Autodesk Fusion 360 part; units mm, degrees
(part 4 of 7)
sketch "Sketch3 (5)" plane through (0, 0, -1.1752) normal (0, 0, 1) x (-1, 0, 0)
  arc A0 (-21.9982, -2.8847) -> (-22.282, -3.9438) centre (-17.5834, -4.6352) ccw
  line L0 (-22.282, -3.9438) -> (-23.1617, -3.816)
  spline S0 degree 5 poles (-23.1617, -3.816) (-23.1657, -3.8154) (-23.1736, -3.8144) (-23.1855, -3.8132) (-23.2015, -3.8124) (-23.2215, -3.8123) (-23.2416, -3.8129) (-23.2618, -3.814) (-23.282, -3.8153) (-23.3022, -3.8168) (-23.3225, -3.8184) (-23.3427, -3.8203) (-23.363, -3.8225) (-23.3833, -3.825) (-23.4037, -3.8279) (-23.424, -3.8311) (-23.4444, -3.8346) (-23.4648, -3.8383) (-23.4852, -3.8422) (-23.5056, -3.8464) (-23.526, -3.8507) (-23.5464, -3.8552) (-23.5669, -3.86) (-23.5873, -3.865) (-23.6077, -3.8702) (-23.6282, -3.8756) (-23.6486, -3.8812) (-23.6691, -3.8871) (-23.6895, -3.8931) (-23.71, -3.8993) (-23.7304, -3.9057) (-23.7509, -3.9123) (-23.7713, -3.919) (-23.7917, -3.926) (-23.8122, -3.9331) (-23.8326, -3.9404) (-23.853, -3.9479) (-23.8734, -3.9556) (-23.8938, -3.9634) (-23.9142, -3.9714) (-23.9345, -3.9796) (-23.9549, -3.988) (-23.9753, -3.9965) (-23.9956, -4.0052) (-24.0159, -4.014) (-24.0362, -4.0231) (-24.0565, -4.0322) (-24.0768, -4.0416) (-24.0971, -4.0511) (-24.1173, -4.0607) (-24.1375, -4.0706) (-24.1577, -4.0805) (-24.1779, -4.0907) (-24.1981, -4.101) (-24.2182, -4.1114) (-24.2384, -4.122) (-24.2585, -4.1327) (-24.2785, -4.1436) (-24.2986, -4.1547) (-24.3186, -4.1659) (-24.3386, -4.1772) (-24.3586, -4.1887) (-24.3786, -4.2004) (-24.3985, -4.2122) (-24.4184, -4.2241) (-24.4383, -4.2362) (-24.4581, -4.2484) (-24.4779, -4.2608) (-24.4977, -4.2733) (-24.5174, -4.286) (-24.5372, -4.2988) (-24.5529, -4.3091) (-24.5647, -4.317) (-24.5726, -4.3222) (-24.5765, -4.3248) knots 0 0 0 0 0 0 0.01428571 0.02857143 0.04285714 0.05714286 0.07142857 0.08571429 0.1 0.11428571 0.12857143 0.14285714 0.15714286 0.17142857 0.18571429 0.2 0.21428571 0.22857143 0.24285714 0.25714286 0.27142857 0.28571429 0.3 0.31428571 0.32857143 0.34285714 0.35714286 0.37142857 0.38571429 0.4 0.41428571 0.42857143 0.44285714 0.45714286 0.47142857 0.48571429 0.5 0.51428571 0.52857143 0.54285714 0.55714286 0.57142857 0.58571429 0.6 0.61428571 0.62857143 0.64285714 0.65714286 0.67142857 0.68571429 0.7 0.71428571 0.72857143 0.74285714 0.75714286 0.77142857 0.78571429 0.8 0.81428571 0.82857143 0.84285714 0.85714286 0.87142857 0.88571429 0.9 0.91428571 0.92857143 0.94285714 0.95714286 0.97142857 0.98571429 1 1 1 1 1 1
  arc A1 (-24.5765, -4.3248) -> (-24.5765, -4.9455) centre (-17.5834, -4.6352) ccw
  spline S1 degree 5 poles (-24.5765, -4.9455) (-24.5726, -4.9482) (-24.5647, -4.9534) (-24.5529, -4.9612) (-24.5372, -4.9716) (-24.5174, -4.9844) (-24.4977, -4.997) (-24.4779, -5.0095) (-24.4581, -5.0219) (-24.4383, -5.0341) (-24.4184, -5.0462) (-24.3985, -5.0582) (-24.3786, -5.07) (-24.3586, -5.0816) (-24.3386, -5.0931) (-24.3186, -5.1044) (-24.2986, -5.1156) (-24.2785, -5.1267) (-24.2585, -5.1376) (-24.2384, -5.1483) (-24.2182, -5.1589) (-24.1981, -5.1694) (-24.1779, -5.1797) (-24.1577, -5.1898) (-24.1375, -5.1998) (-24.1173, -5.2096) (-24.0971, -5.2193) (-24.0768, -5.2288) (-24.0565, -5.2381) (-24.0362, -5.2473) (-24.0159, -5.2563) (-23.9956, -5.2652) (-23.9753, -5.2738) (-23.9549, -5.2824) (-23.9345, -5.2907) (-23.9142, -5.2989) (-23.8938, -5.3069) (-23.8734, -5.3148) (-23.853, -5.3224) (-23.8326, -5.3299) (-23.8122, -5.3372) (-23.7917, -5.3444) (-23.7713, -5.3513) (-23.7509, -5.3581) (-23.7304, -5.3647) (-23.71, -5.3711) (-23.6895, -5.3773) (-23.6691, -5.3833) (-23.6486, -5.3891) (-23.6282, -5.3947) (-23.6077, -5.4002) (-23.5873, -5.4054) (-23.5669, -5.4104) (-23.5464, -5.4151) (-23.526, -5.4197) (-23.5056, -5.424) (-23.4852, -5.4281) (-23.4648, -5.4321) (-23.4444, -5.4358) (-23.424, -5.4393) (-23.4037, -5.4425) (-23.3833, -5.4454) (-23.363, -5.4479) (-23.3427, -5.4501) (-23.3225, -5.4519) (-23.3022, -5.4536) (-23.282, -5.4551) (-23.2618, -5.4564) (-23.2416, -5.4574) (-23.2215, -5.458) (-23.2015, -5.458) (-23.1855, -5.4571) (-23.1736, -5.4559) (-23.1657, -5.4549) (-23.1617, -5.4543) knots -1 -1 -1 -1 -1 -1 -0.98571429 -0.97142857 -0.95714286 -0.94285714 -0.92857143 -0.91428571 -0.9 -0.88571429 -0.87142857 -0.85714286 -0.84285714 -0.82857143 -0.81428571 -0.8 -0.78571429 -0.77142857 -0.75714286 -0.74285714 -0.72857143 -0.71428571 -0.7 -0.68571429 -0.67142857 -0.65714286 -0.64285714 -0.62857143 -0.61428571 -0.6 -0.58571429 -0.57142857 -0.55714286 -0.54285714 -0.52857143 -0.51428571 -0.5 -0.48571429 -0.47142857 -0.45714286 -0.44285714 -0.42857143 -0.41428571 -0.4 -0.38571429 -0.37142857 -0.35714286 -0.34285714 -0.32857143 -0.31428571 -0.3 -0.28571429 -0.27142857 -0.25714286 -0.24285714 -0.22857143 -0.21428571 -0.2 -0.18571429 -0.17142857 -0.15714286 -0.14285714 -0.12857143 -0.11428571 -0.1 -0.08571429 -0.07142857 -0.05714286 -0.04285714 -0.02857143 -0.01428571 0 0 0 0 0 0
  line L1 (-23.1617, -5.4543) -> (-22.282, -5.3266)
  arc A2 (-22.282, -5.3266) -> (-21.9982, -6.3857) centre (-17.5834, -4.6352) ccw
  line L2 (-21.9982, -6.3857) -> (-22.8239, -6.7149)
  spline S2 degree 5 poles (-22.8239, -6.7149) (-22.8277, -6.7164) (-22.835, -6.7195) (-22.8459, -6.7244) (-22.8602, -6.7317) (-22.8776, -6.7416) (-22.8947, -6.7522) (-22.9116, -6.7632) (-22.9285, -6.7744) (-22.9452, -6.7858) (-22.9619, -6.7974) (-22.9786, -6.8091) (-22.995, -6.8212) (-23.0114, -6.8335) (-23.0275, -6.8462) (-23.0436, -6.8591) (-23.0595, -6.8723) (-23.0753, -6.8857) (-23.091, -6.8994) (-23.1066, -6.9131) (-23.1221, -6.9271) (-23.1375, -6.9412) (-23.1528, -6.9556) (-23.168, -6.9701) (-23.1831, -6.9849) (-23.1981, -6.9998) (-23.213, -7.0149) (-23.2278, -7.0301) (-23.2425, -7.0456) (-23.2571, -7.0612) (-23.2716, -7.0769) (-23.286, -7.0929) (-23.3003, -7.1089) (-23.3146, -7.1252) (-23.3287, -7.1416) (-23.3427, -7.1581) (-23.3566, -7.1748) (-23.3705, -7.1916) (-23.3842, -7.2086) (-23.3979, -7.2258) (-23.4114, -7.243) (-23.4249, -7.2605) (-23.4382, -7.278) (-23.4515, -7.2957) (-23.4647, -7.3135) (-23.4778, -7.3315) (-23.4907, -7.3496) (-23.5036, -7.3678) (-23.5164, -7.3862) (-23.5291, -7.4047) (-23.5417, -7.4233) (-23.5543, -7.442) (-23.5667, -7.4609) (-23.579, -7.4799) (-23.5912, -7.499) (-23.6033, -7.5182) (-23.6154, -7.5376) (-23.6273, -7.5571) (-23.6392, -7.5767) (-23.6509, -7.5964) (-23.6626, -7.6162) (-23.6741, -7.6362) (-23.6856, -7.6562) (-23.6969, -7.6764) (-23.7082, -7.6967) (-23.7194, -7.7171) (-23.7304, -7.7376) (-23.7414, -7.7582) (-23.7523, -7.7789) (-23.7631, -7.7998) (-23.7737, -7.8207) (-23.7822, -7.8376) (-23.7885, -7.8502) (-23.7927, -7.8587) (-23.7948, -7.863) knots 0 0 0 0 0 0 0.01428571 0.02857143 0.04285714 0.05714286 0.07142857 0.08571429 0.1 0.11428571 0.12857143 0.14285714 0.15714286 0.17142857 0.18571429 0.2 0.21428571 0.22857143 0.24285714 0.25714286 0.27142857 0.28571429 0.3 0.31428571 0.32857143 0.34285714 0.35714286 0.37142857 0.38571429 0.4 0.41428571 0.42857143 0.44285714 0.45714286 0.47142857 0.48571429 0.5 0.51428571 0.52857143 0.54285714 0.55714286 0.57142857 0.58571429 0.6 0.61428571 0.62857143 0.64285714 0.65714286 0.67142857 0.68571429 0.7 0.71428571 0.72857143 0.74285714 0.75714286 0.77142857 0.78571429 0.8 0.81428571 0.82857143 0.84285714 0.85714286 0.87142857 0.88571429 0.9 0.91428571 0.92857143 0.94285714 0.95714286 0.97142857 0.98571429 1 1 1 1 1 1
  arc A3 (-23.7948, -7.863) -> (-23.4844, -8.4005) centre (-17.5834, -4.6352) ccw
  spline S3 degree 5 poles (-23.4844, -8.4005) (-23.4797, -8.4008) (-23.4703, -8.4014) (-23.4561, -8.4023) (-23.4373, -8.4034) (-23.4139, -8.4046) (-23.3904, -8.4057) (-23.367, -8.4067) (-23.3437, -8.4075) (-23.3204, -8.4081) (-23.2971, -8.4087) (-23.2739, -8.409) (-23.2508, -8.4093) (-23.2277, -8.4094) (-23.2046, -8.4094) (-23.1816, -8.4092) (-23.1587, -8.4089) (-23.1358, -8.4084) (-23.113, -8.4078) (-23.0902, -8.4071) (-23.0674, -8.4062) (-23.0448, -8.4052) (-23.0222, -8.404) (-22.9996, -8.4027) (-22.9771, -8.4012) (-22.9547, -8.3996) (-22.9323, -8.3978) (-22.91, -8.3959) (-22.8878, -8.3939) (-22.8657, -8.3917) (-22.8436, -8.3894) (-22.8215, -8.3869) (-22.7996, -8.3842) (-22.7777, -8.3814) (-22.7559, -8.3785) (-22.7341, -8.3754) (-22.7125, -8.3721) (-22.6909, -8.3687) (-22.6694, -8.3652) (-22.648, -8.3614) (-22.6266, -8.3576) (-22.6054, -8.3535) (-22.5842, -8.3493) (-22.5631, -8.345) (-22.5421, -8.3404) (-22.5212, -8.3358) (-22.5004, -8.3309) (-22.4797, -8.3259) (-22.4591, -8.3207) (-22.4386, -8.3154) (-22.4181, -8.3099) (-22.3978, -8.3042) (-22.3776, -8.2983) (-22.3576, -8.2922) (-22.3376, -8.2859) (-22.3178, -8.2794) (-22.298, -8.2728) (-22.2784, -8.266) (-22.2589, -8.259) (-22.2395, -8.2519) (-22.2202, -8.2445) (-22.2012, -8.2368) (-22.1823, -8.2288) (-22.1637, -8.2206) (-22.1452, -8.2121) (-22.1268, -8.2034) (-22.1086, -8.1945) (-22.0904, -8.1856) (-22.0724, -8.1764) (-22.0547, -8.1669) (-22.0374, -8.1568) (-22.024, -8.1481) (-22.0143, -8.1411) (-22.0079, -8.1362) (-22.0048, -8.1338) knots -1 -1 -1 -1 -1 -1 -0.98571429 -0.97142857 -0.95714286 -0.94285714 -0.92857143 -0.91428571 -0.9 -0.88571429 -0.87142857 -0.85714286 -0.84285714 -0.82857143 -0.81428571 -0.8 -0.78571429 -0.77142857 -0.75714286 -0.74285714 -0.72857143 -0.71428571 -0.7 -0.68571429 -0.67142857 -0.65714286 -0.64285714 -0.62857143 -0.61428571 -0.6 -0.58571429 -0.57142857 -0.55714286 -0.54285714 -0.52857143 -0.51428571 -0.5 -0.48571429 -0.47142857 -0.45714286 -0.44285714 -0.42857143 -0.41428571 -0.4 -0.38571429 -0.37142857 -0.35714286 -0.34285714 -0.32857143 -0.31428571 -0.3 -0.28571429 -0.27142857 -0.25714286 -0.24285714 -0.22857143 -0.21428571 -0.2 -0.18571429 -0.17142857 -0.15714286 -0.14285714 -0.12857143 -0.11428571 -0.1 -0.08571429 -0.07142857 -0.05714286 -0.04285714 -0.02857143 -0.01428571 0 0 0 0 0 0
  line L3 (-22.0048, -8.1338) -> (-21.3068, -7.5833)
  arc A4 (-21.3068, -7.5833) -> (-20.5315, -8.3586) centre (-17.5834, -4.6352) ccw
  line L4 (-20.5315, -8.3586) -> (-21.082, -9.0566)
  spline S4 degree 5 poles (-21.082, -9.0566) (-21.0844, -9.0597) (-21.0893, -9.0661) (-21.0963, -9.0758) (-21.105, -9.0892) (-21.1151, -9.1065) (-21.1246, -9.1242) (-21.1338, -9.1422) (-21.1427, -9.1604) (-21.1516, -9.1786) (-21.1603, -9.197) (-21.1688, -9.2155) (-21.177, -9.2341) (-21.185, -9.253) (-21.1927, -9.272) (-21.2001, -9.2913) (-21.2072, -9.3107) (-21.2142, -9.3302) (-21.221, -9.3498) (-21.2276, -9.3696) (-21.2341, -9.3894) (-21.2404, -9.4094) (-21.2465, -9.4294) (-21.2524, -9.4496) (-21.2581, -9.4699) (-21.2636, -9.4903) (-21.2689, -9.5109) (-21.2741, -9.5315) (-21.2791, -9.5522) (-21.284, -9.573) (-21.2887, -9.5939) (-21.2932, -9.6149) (-21.2975, -9.636) (-21.3017, -9.6572) (-21.3058, -9.6784) (-21.3096, -9.6998) (-21.3134, -9.7212) (-21.3169, -9.7427) (-21.3203, -9.7643) (-21.3236, -9.7859) (-21.3267, -9.8077) (-21.3296, -9.8295) (-21.3324, -9.8514) (-21.3351, -9.8733) (-21.3376, -9.8953) (-21.3399, -9.9174) (-21.3421, -9.9396) (-21.3442, -9.9618) (-21.3461, -9.9841) (-21.3478, -10.0065) (-21.3494, -10.0289) (-21.3509, -10.0514) (-21.3522, -10.074) (-21.3534, -10.0966) (-21.3544, -10.1192) (-21.3553, -10.142) (-21.356, -10.1647) (-21.3566, -10.1876) (-21.3571, -10.2105) (-21.3574, -10.2334) (-21.3576, -10.2564) (-21.3576, -10.2795) (-21.3575, -10.3026) (-21.3573, -10.3257) (-21.3569, -10.3489) (-21.3563, -10.3722) (-21.3557, -10.3955) (-21.3549, -10.4188) (-21.3539, -10.4422) (-21.3528, -10.4656) (-21.3516, -10.4891) (-21.3505, -10.5079) (-21.3496, -10.5221) (-21.349, -10.5315) (-21.3487, -10.5362) knots 0 0 0 0 0 0 0.01428571 0.02857143 0.04285714 0.05714286 0.07142857 0.08571429 0.1 0.11428571 0.12857143 0.14285714 0.15714286 0.17142857 0.18571429 0.2 0.21428571 0.22857143 0.24285714 0.25714286 0.27142857 0.28571429 0.3 0.31428571 0.32857143 0.34285714 0.35714286 0.37142857 0.38571429 0.4 0.41428571 0.42857143 0.44285714 0.45714286 0.47142857 0.48571429 0.5 0.51428571 0.52857143 0.54285714 0.55714286 0.57142857 0.58571429 0.6 0.61428571 0.62857143 0.64285714 0.65714286 0.67142857 0.68571429 0.7 0.71428571 0.72857143 0.74285714 0.75714286 0.77142857 0.78571429 0.8 0.81428571 0.82857143 0.84285714 0.85714286 0.87142857 0.88571429 0.9 0.91428571 0.92857143 0.94285714 0.95714286 0.97142857 0.98571429 1 1 1 1 1 1
  arc A5 (-21.3487, -10.5362) -> (-20.8112, -10.8466) centre (-17.5834, -4.6352) ccw
  spline S5 degree 5 poles (-20.8112, -10.8466) (-20.8069, -10.8445) (-20.7985, -10.8403) (-20.7858, -10.834) (-20.7689, -10.8255) (-20.748, -10.8148) (-20.7272, -10.8041) (-20.7064, -10.7932) (-20.6858, -10.7822) (-20.6653, -10.7712) (-20.6449, -10.76) (-20.6246, -10.7487) (-20.6044, -10.7374) (-20.5844, -10.7259) (-20.5644, -10.7143) (-20.5446, -10.7027) (-20.5249, -10.6909) (-20.5053, -10.6791) (-20.4858, -10.6672) (-20.4664, -10.6551) (-20.4472, -10.643) (-20.4281, -10.6308) (-20.4091, -10.6185) (-20.3902, -10.606) (-20.3715, -10.5935) (-20.3529, -10.5809) (-20.3344, -10.5682) (-20.316, -10.5554) (-20.2978, -10.5425) (-20.2797, -10.5296) (-20.2617, -10.5165) (-20.2439, -10.5033) (-20.2262, -10.49) (-20.2087, -10.4767) (-20.1912, -10.4632) (-20.174, -10.4497) (-20.1568, -10.436) (-20.1398, -10.4223) (-20.123, -10.4084) (-20.1063, -10.3945) (-20.0898, -10.3805) (-20.0734, -10.3664) (-20.0571, -10.3521) (-20.0411, -10.3378) (-20.0251, -10.3234) (-20.0094, -10.3089) (-19.9938, -10.2943) (-19.9784, -10.2796) (-19.9631, -10.2648) (-19.948, -10.2499) (-19.9331, -10.2349) (-19.9183, -10.2198) (-19.9038, -10.2046) (-19.8895, -10.1893) (-19.8753, -10.1739) (-19.8613, -10.1584) (-19.8476, -10.1428) (-19.834, -10.1271) (-19.8205, -10.1113) (-19.8073, -10.0954) (-19.7944, -10.0793) (-19.7817, -10.0632) (-19.7694, -10.0468) (-19.7573, -10.0304) (-19.7456, -10.0137) (-19.734, -9.997) (-19.7226, -9.9803) (-19.7114, -9.9634) (-19.7004, -9.9465) (-19.6898, -9.9294) (-19.6799, -9.912) (-19.6726, -9.8977) (-19.6677, -9.8868) (-19.6646, -9.8794) (-19.6631, -9.8757) knots -1 -1 -1 -1 -1 -1 -0.98571429 -0.97142857 -0.95714286 -0.94285714 -0.92857143 -0.91428571 -0.9 -0.88571429 -0.87142857 -0.85714286 -0.84285714 -0.82857143 -0.81428571 -0.8 -0.78571429 -0.77142857 -0.75714286 -0.74285714 -0.72857143 -0.71428571 -0.7 -0.68571429 -0.67142857 -0.65714286 -0.64285714 -0.62857143 -0.61428571 -0.6 -0.58571429 -0.57142857 -0.55714286 -0.54285714 -0.52857143 -0.51428571 -0.5 -0.48571429 -0.47142857 -0.45714286 -0.44285714 -0.42857143 -0.41428571 -0.4 -0.38571429 -0.37142857 -0.35714286 -0.34285714 -0.32857143 -0.31428571 -0.3 -0.28571429 -0.27142857 -0.25714286 -0.24285714 -0.22857143 -0.21428571 -0.2 -0.18571429 -0.17142857 -0.15714286 -0.14285714 -0.12857143 -0.11428571 -0.1 -0.08571429 -0.07142857 -0.05714286 -0.04285714 -0.02857143 -0.01428571 0 0 0 0 0 0
  line L5 (-19.6631, -9.8757) -> (-19.3339, -9.05)
  arc A6 (-19.3339, -9.05) -> (-18.2748, -9.3338) centre (-17.5834, -4.6352) ccw
  line L6 (-18.2748, -9.3338) -> (-18.4025, -10.2135)
  spline S6 degree 5 poles (-18.4025, -10.2135) (-18.4031, -10.2175) (-18.4041, -10.2254) (-18.4053, -10.2373) (-18.4062, -10.2533) (-18.4063, -10.2733) (-18.4056, -10.2934) (-18.4046, -10.3136) (-18.4033, -10.3338) (-18.4018, -10.354) (-18.4001, -10.3742) (-18.3983, -10.3945) (-18.3961, -10.4148) (-18.3936, -10.4351) (-18.3907, -10.4555) (-18.3875, -10.4758) (-18.384, -10.4962) (-18.3803, -10.5166) (-18.3763, -10.537) (-18.3722, -10.5574) (-18.3679, -10.5778) (-18.3633, -10.5982) (-18.3586, -10.6187) (-18.3536, -10.6391) (-18.3484, -10.6595) (-18.343, -10.68) (-18.3373, -10.7004) (-18.3315, -10.7209) (-18.3255, -10.7413) (-18.3193, -10.7618) (-18.3129, -10.7822) (-18.3063, -10.8027) (-18.2995, -10.8231) (-18.2926, -10.8435) (-18.2854, -10.8639) (-18.2781, -10.8844) (-18.2706, -10.9048) (-18.263, -10.9252) (-18.2551, -10.9456) (-18.2471, -10.966) (-18.2389, -10.9863) (-18.2306, -11.0067) (-18.2221, -11.027) (-18.2134, -11.0474) (-18.2045, -11.0677) (-18.1955, -11.088) (-18.1863, -11.1083) (-18.177, -11.1286) (-18.1675, -11.1488) (-18.1578, -11.1691) (-18.148, -11.1893) (-18.138, -11.2095) (-18.1279, -11.2297) (-18.1176, -11.2499) (-18.1072, -11.27) (-18.0966, -11.2901) (-18.0858, -11.3102) (-18.0749, -11.3303) (-18.0639, -11.3504) (-18.0527, -11.3704) (-18.0413, -11.3904) (-18.0298, -11.4104) (-18.0182, -11.4303) (-18.0064, -11.4503) (-17.9944, -11.4702) (-17.9824, -11.49) (-17.9701, -11.5099) (-17.9578, -11.5297) (-17.9452, -11.5495) (-17.9326, -11.5692) (-17.9198, -11.589) (-17.9094, -11.6047) (-17.9016, -11.6165) (-17.8964, -11.6244) (-17.8937, -11.6283) knots 0 0 0 0 0 0 0.01428571 0.02857143 0.04285714 0.05714286 0.07142857 0.08571429 0.1 0.11428571 0.12857143 0.14285714 0.15714286 0.17142857 0.18571429 0.2 0.21428571 0.22857143 0.24285714 0.25714286 0.27142857 0.28571429 0.3 0.31428571 0.32857143 0.34285714 0.35714286 0.37142857 0.38571429 0.4 0.41428571 0.42857143 0.44285714 0.45714286 0.47142857 0.48571429 0.5 0.51428571 0.52857143 0.54285714 0.55714286 0.57142857 0.58571429 0.6 0.61428571 0.62857143 0.64285714 0.65714286 0.67142857 0.68571429 0.7 0.71428571 0.72857143 0.74285714 0.75714286 0.77142857 0.78571429 0.8 0.81428571 0.82857143 0.84285714 0.85714286 0.87142857 0.88571429 0.9 0.91428571 0.92857143 0.94285714 0.95714286 0.97142857 0.98571429 1 1 1 1 1 1
  arc A7 (-17.8937, -11.6283) -> (-17.273, -11.6283) centre (-17.5834, -4.6352) ccw
  spline S7 degree 5 poles (-17.273, -11.6283) (-17.2704, -11.6244) (-17.2652, -11.6165) (-17.2573, -11.6047) (-17.247, -11.589) (-17.2342, -11.5692) (-17.2215, -11.5495) (-17.209, -11.5297) (-17.1966, -11.5099) (-17.1844, -11.49) (-17.1723, -11.4702) (-17.1604, -11.4503) (-17.1486, -11.4303) (-17.137, -11.4104) (-17.1255, -11.3904) (-17.1141, -11.3704) (-17.1029, -11.3504) (-17.0919, -11.3303) (-17.081, -11.3102) (-17.0702, -11.2901) (-17.0596, -11.27) (-17.0492, -11.2499) (-17.0389, -11.2297) (-17.0288, -11.2095) (-17.0188, -11.1893) (-17.009, -11.1691) (-16.9993, -11.1488) (-16.9898, -11.1286) (-16.9804, -11.1083) (-16.9713, -11.088) (-16.9623, -11.0677) (-16.9534, -11.0474) (-16.9447, -11.027) (-16.9362, -11.0067) (-16.9278, -10.9863) (-16.9197, -10.966) (-16.9116, -10.9456) (-16.9038, -10.9252) (-16.8961, -10.9048) (-16.8886, -10.8844) (-16.8813, -10.8639) (-16.8742, -10.8435) (-16.8672, -10.8231) (-16.8605, -10.8027) (-16.8539, -10.7822) (-16.8475, -10.7618) (-16.8413, -10.7413) (-16.8353, -10.7209) (-16.8294, -10.7004) (-16.8238, -10.68) (-16.8184, -10.6595) (-16.8132, -10.6391) (-16.8082, -10.6187) (-16.8034, -10.5982) (-16.7989, -10.5778) (-16.7946, -10.5574) (-16.7904, -10.537) (-16.7865, -10.5166) (-16.7828, -10.4962) (-16.7793, -10.4758) (-16.7761, -10.4555) (-16.7732, -10.4351) (-16.7707, -10.4148) (-16.7685, -10.3945) (-16.7666, -10.3742) (-16.765, -10.354) (-16.7635, -10.3338) (-16.7622, -10.3136) (-16.7611, -10.2934) (-16.7605, -10.2733) (-16.7606, -10.2533) (-16.7615, -10.2373) (-16.7626, -10.2254) (-16.7637, -10.2175) (-16.7642, -10.2135) knots -1 -1 -1 -1 -1 -1 -0.98571429 -0.97142857 -0.95714286 -0.94285714 -0.92857143 -0.91428571 -0.9 -0.88571429 -0.87142857 -0.85714286 -0.84285714 -0.82857143 -0.81428571 -0.8 -0.78571429 -0.77142857 -0.75714286 -0.74285714 -0.72857143 -0.71428571 -0.7 -0.68571429 -0.67142857 -0.65714286 -0.64285714 -0.62857143 -0.61428571 -0.6 -0.58571429 -0.57142857 -0.55714286 -0.54285714 -0.52857143 -0.51428571 -0.5 -0.48571429 -0.47142857 -0.45714286 -0.44285714 -0.42857143 -0.41428571 -0.4 -0.38571429 -0.37142857 -0.35714286 -0.34285714 -0.32857143 -0.31428571 -0.3 -0.28571429 -0.27142857 -0.25714286 -0.24285714 -0.22857143 -0.21428571 -0.2 -0.18571429 -0.17142857 -0.15714286 -0.14285714 -0.12857143 -0.11428571 -0.1 -0.08571429 -0.07142857 -0.05714286 -0.04285714 -0.02857143 -0.01428571 0 0 0 0 0 0
  line L7 (-16.7642, -10.2135) -> (-16.892, -9.3338)
  arc A8 (-16.892, -9.3338) -> (-15.8329, -9.05) centre (-17.5834, -4.6352) ccw
  line L8 (-15.8329, -9.05) -> (-15.5036, -9.8757)
  spline S8 degree 5 poles (-15.5036, -9.8757) (-15.5021, -9.8794) (-15.4991, -9.8868) (-15.4941, -9.8977) (-15.4869, -9.912) (-15.4769, -9.9294) (-15.4663, -9.9465) (-15.4554, -9.9634) (-15.4441, -9.9803) (-15.4327, -9.997) (-15.4212, -10.0137) (-15.4094, -10.0304) (-15.3974, -10.0468) (-15.385, -10.0632) (-15.3724, -10.0793) (-15.3594, -10.0954) (-15.3462, -10.1113) (-15.3328, -10.1271) (-15.3192, -10.1428) (-15.3054, -10.1584) (-15.2915, -10.1739) (-15.2773, -10.1893) (-15.263, -10.2046) (-15.2484, -10.2198) (-15.2337, -10.2349) (-15.2188, -10.2499) (-15.2037, -10.2648) (-15.1884, -10.2796) (-15.173, -10.2943) (-15.1574, -10.3089) (-15.1416, -10.3234) (-15.1257, -10.3378) (-15.1096, -10.3521) (-15.0934, -10.3664) (-15.077, -10.3805) (-15.0605, -10.3945) (-15.0438, -10.4084) (-15.0269, -10.4223) (-15.0099, -10.436) (-14.9928, -10.4497) (-14.9755, -10.4632) (-14.9581, -10.4767) (-14.9406, -10.49) (-14.9229, -10.5033) (-14.905, -10.5165) (-14.8871, -10.5296) (-14.869, -10.5425) (-14.8507, -10.5554) (-14.8324, -10.5682) (-14.8139, -10.5809) (-14.7953, -10.5935) (-14.7765, -10.606) (-14.7577, -10.6185) (-14.7387, -10.6308) (-14.7196, -10.643) (-14.7003, -10.6551) (-14.681, -10.6672) (-14.6615, -10.6791) (-14.6419, -10.6909) (-14.6222, -10.7027) (-14.6023, -10.7143) (-14.5824, -10.7259) (-14.5623, -10.7374) (-14.5422, -10.7487) (-14.5219, -10.76) (-14.5015, -10.7712) (-14.481, -10.7822) (-14.4603, -10.7932) (-14.4396, -10.8041) (-14.4188, -10.8148) (-14.3978, -10.8255) (-14.381, -10.834) (-14.3683, -10.8403) (-14.3598, -10.8445) (-14.3556, -10.8466) knots 0 0 0 0 0 0 0.01428571 0.02857143 0.04285714 0.05714286 0.07142857 0.08571429 0.1 0.11428571 0.12857143 0.14285714 0.15714286 0.17142857 0.18571429 0.2 0.21428571 0.22857143 0.24285714 0.25714286 0.27142857 0.28571429 0.3 0.31428571 0.32857143 0.34285714 0.35714286 0.37142857 0.38571429 0.4 0.41428571 0.42857143 0.44285714 0.45714286 0.47142857 0.48571429 0.5 0.51428571 0.52857143 0.54285714 0.55714286 0.57142857 0.58571429 0.6 0.61428571 0.62857143 0.64285714 0.65714286 0.67142857 0.68571429 0.7 0.71428571 0.72857143 0.74285714 0.75714286 0.77142857 0.78571429 0.8 0.81428571 0.82857143 0.84285714 0.85714286 0.87142857 0.88571429 0.9 0.91428571 0.92857143 0.94285714 0.95714286 0.97142857 0.98571429 1 1 1 1 1 1
  arc A9 (-14.3556, -10.8466) -> (-13.8181, -10.5362) centre (-17.5834, -4.6352) ccw
  spline S9 degree 5 poles (-13.8181, -10.5362) (-13.8177, -10.5315) (-13.8171, -10.5221) (-13.8162, -10.5079) (-13.8152, -10.4891) (-13.8139, -10.4656) (-13.8129, -10.4422) (-13.8119, -10.4188) (-13.8111, -10.3955) (-13.8104, -10.3722) (-13.8099, -10.3489) (-13.8095, -10.3257) (-13.8093, -10.3026) (-13.8092, -10.2795) (-13.8092, -10.2564) (-13.8094, -10.2334) (-13.8097, -10.2105) (-13.8101, -10.1876) (-13.8107, -10.1647) (-13.8115, -10.142) (-13.8124, -10.1192) (-13.8134, -10.0966) (-13.8146, -10.074) (-13.8159, -10.0514) (-13.8173, -10.0289) (-13.819, -10.0065) (-13.8207, -9.9841) (-13.8226, -9.9618) (-13.8247, -9.9396) (-13.8269, -9.9174) (-13.8292, -9.8953) (-13.8317, -9.8733) (-13.8343, -9.8514) (-13.8371, -9.8295) (-13.8401, -9.8077) (-13.8432, -9.7859) (-13.8464, -9.7643) (-13.8498, -9.7427) (-13.8534, -9.7212) (-13.8571, -9.6998) (-13.861, -9.6784) (-13.865, -9.6572) (-13.8692, -9.636) (-13.8736, -9.6149) (-13.8781, -9.5939) (-13.8828, -9.573) (-13.8876, -9.5522) (-13.8927, -9.5315) (-13.8978, -9.5109) (-13.9032, -9.4903) (-13.9087, -9.4699) (-13.9144, -9.4496) (-13.9203, -9.4294) (-13.9264, -9.4094) (-13.9327, -9.3894) (-13.9391, -9.3696) (-13.9458, -9.3498) (-13.9526, -9.3302) (-13.9595, -9.3107) (-13.9667, -9.2913) (-13.9741, -9.272) (-13.9818, -9.253) (-13.9897, -9.2341) (-13.998, -9.2155) (-14.0065, -9.197) (-14.0152, -9.1786) (-14.024, -9.1604) (-14.033, -9.1422) (-14.0422, -9.1242) (-14.0517, -9.1065) (-14.0618, -9.0892) (-14.0705, -9.0758) (-14.0775, -9.0661) (-14.0823, -9.0597) (-14.0848, -9.0566) knots -1 -1 -1 -1 -1 -1 -0.98571429 -0.97142857 -0.95714286 -0.94285714 -0.92857143 -0.91428571 -0.9 -0.88571429 -0.87142857 -0.85714286 -0.84285714 -0.82857143 -0.81428571 -0.8 -0.78571429 -0.77142857 -0.75714286 -0.74285714 -0.72857143 -0.71428571 -0.7 -0.68571429 -0.67142857 -0.65714286 -0.64285714 -0.62857143 -0.61428571 -0.6 -0.58571429 -0.57142857 -0.55714286 -0.54285714 -0.52857143 -0.51428571 -0.5 -0.48571429 -0.47142857 -0.45714286 -0.44285714 -0.42857143 -0.41428571 -0.4 -0.38571429 -0.37142857 -0.35714286 -0.34285714 -0.32857143 -0.31428571 -0.3 -0.28571429 -0.27142857 -0.25714286 -0.24285714 -0.22857143 -0.21428571 -0.2 -0.18571429 -0.17142857 -0.15714286 -0.14285714 -0.12857143 -0.11428571 -0.1 -0.08571429 -0.07142857 -0.05714286 -0.04285714 -0.02857143 -0.01428571 0 0 0 0 0 0
  line L9 (-14.0848, -9.0566) -> (-14.6353, -8.3586)
  arc A10 (-14.6353, -8.3586) -> (-13.86, -7.5833) centre (-17.5834, -4.6352) ccw
  line L10 (-13.86, -7.5833) -> (-13.162, -8.1338)
  spline S10 degree 5 poles (-13.162, -8.1338) (-13.1588, -8.1362) (-13.1525, -8.1411) (-13.1427, -8.1481) (-13.1293, -8.1568) (-13.112, -8.1669) (-13.0943, -8.1764) (-13.0763, -8.1856) (-13.0582, -8.1945) (-13.0399, -8.2034) (-13.0216, -8.2121) (-13.0031, -8.2206) (-12.9844, -8.2288) (-12.9656, -8.2368) (-12.9465, -8.2445) (-12.9273, -8.2519) (-12.9079, -8.259) (-12.8884, -8.266) (-12.8687, -8.2728) (-12.849, -8.2794) (-12.8292, -8.2859) (-12.8092, -8.2922) (-12.7891, -8.2983) (-12.7689, -8.3042) (-12.7486, -8.3099) (-12.7282, -8.3154) (-12.7077, -8.3207) (-12.6871, -8.3259) (-12.6663, -8.3309) (-12.6455, -8.3358) (-12.6246, -8.3404) (-12.6036, -8.345) (-12.5826, -8.3493) (-12.5614, -8.3535) (-12.5401, -8.3576) (-12.5188, -8.3614) (-12.4974, -8.3652) (-12.4759, -8.3687) (-12.4543, -8.3721) (-12.4326, -8.3754) (-12.4109, -8.3785) (-12.3891, -8.3814) (-12.3672, -8.3842) (-12.3452, -8.3869) (-12.3232, -8.3894) (-12.3011, -8.3917) (-12.279, -8.3939) (-12.2567, -8.3959) (-12.2344, -8.3978) (-12.2121, -8.3996) (-12.1896, -8.4012) (-12.1671, -8.4027) (-12.1446, -8.404) (-12.122, -8.4052) (-12.0993, -8.4062) (-12.0766, -8.4071) (-12.0538, -8.4078) (-12.031, -8.4084) (-12.0081, -8.4089) (-11.9851, -8.4092) (-11.9621, -8.4094) (-11.9391, -8.4094) (-11.916, -8.4093) (-11.8928, -8.409) (-11.8696, -8.4087) (-11.8464, -8.4081) (-11.8231, -8.4075) (-11.7997, -8.4067) (-11.7763, -8.4057) (-11.7529, -8.4046) (-11.7294, -8.4034) (-11.7106, -8.4023) (-11.6965, -8.4014) (-11.6871, -8.4008) (-11.6823, -8.4005) knots 0 0 0 0 0 0 0.01428571 0.02857143 0.04285714 0.05714286 0.07142857 0.08571429 0.1 0.11428571 0.12857143 0.14285714 0.15714286 0.17142857 0.18571429 0.2 0.21428571 0.22857143 0.24285714 0.25714286 0.27142857 0.28571429 0.3 0.31428571 0.32857143 0.34285714 0.35714286 0.37142857 0.38571429 0.4 0.41428571 0.42857143 0.44285714 0.45714286 0.47142857 0.48571429 0.5 0.51428571 0.52857143 0.54285714 0.55714286 0.57142857 0.58571429 0.6 0.61428571 0.62857143 0.64285714 0.65714286 0.67142857 0.68571429 0.7 0.71428571 0.72857143 0.74285714 0.75714286 0.77142857 0.78571429 0.8 0.81428571 0.82857143 0.84285714 0.85714286 0.87142857 0.88571429 0.9 0.91428571 0.92857143 0.94285714 0.95714286 0.97142857 0.98571429 1 1 1 1 1 1
  arc A11 (-11.6823, -8.4005) -> (-11.372, -7.863) centre (-17.5834, -4.6352) ccw
  spline S11 degree 5 poles (-11.372, -7.863) (-11.3741, -7.8587) (-11.3783, -7.8502) (-11.3846, -7.8376) (-11.393, -7.8207) (-11.4037, -7.7998) (-11.4145, -7.7789) (-11.4254, -7.7582) (-11.4363, -7.7376) (-11.4474, -7.7171) (-11.4586, -7.6967) (-11.4698, -7.6764) (-11.4812, -7.6562) (-11.4927, -7.6362) (-11.5042, -7.6162) (-11.5159, -7.5964) (-11.5276, -7.5767) (-11.5395, -7.5571) (-11.5514, -7.5376) (-11.5634, -7.5182) (-11.5756, -7.499) (-11.5878, -7.4799) (-11.6001, -7.4609) (-11.6125, -7.442) (-11.625, -7.4233) (-11.6376, -7.4047) (-11.6503, -7.3862) (-11.6631, -7.3678) (-11.676, -7.3496) (-11.689, -7.3315) (-11.7021, -7.3135) (-11.7153, -7.2957) (-11.7285, -7.278) (-11.7419, -7.2605) (-11.7553, -7.243) (-11.7689, -7.2258) (-11.7825, -7.2086) (-11.7963, -7.1916) (-11.8101, -7.1748) (-11.8241, -7.1581) (-11.8381, -7.1416) (-11.8522, -7.1252) (-11.8664, -7.1089) (-11.8807, -7.0929) (-11.8952, -7.0769) (-11.9097, -7.0612) (-11.9243, -7.0456) (-11.939, -7.0301) (-11.9538, -7.0149) (-11.9686, -6.9998) (-11.9836, -6.9849) (-11.9987, -6.9701) (-12.0139, -6.9556) (-12.0293, -6.9412) (-12.0447, -6.9271) (-12.0602, -6.9131) (-12.0758, -6.8994) (-12.0915, -6.8857) (-12.1073, -6.8723) (-12.1232, -6.8591) (-12.1392, -6.8462) (-12.1554, -6.8335) (-12.1717, -6.8212) (-12.1882, -6.8091) (-12.2048, -6.7974) (-12.2215, -6.7858) (-12.2383, -6.7744) (-12.2551, -6.7632) (-12.2721, -6.7522) (-12.2892, -6.7416) (-12.3066, -6.7317) (-12.3208, -6.7244) (-12.3317, -6.7195) (-12.3391, -6.7164) (-12.3428, -6.7149) knots -1 -1 -1 -1 -1 -1 -0.98571429 -0.97142857 -0.95714286 -0.94285714 -0.92857143 -0.91428571 -0.9 -0.88571429 -0.87142857 -0.85714286 -0.84285714 -0.82857143 -0.81428571 -0.8 -0.78571429 -0.77142857 -0.75714286 -0.74285714 -0.72857143 -0.71428571 -0.7 -0.68571429 -0.67142857 -0.65714286 -0.64285714 -0.62857143 -0.61428571 -0.6 -0.58571429 -0.57142857 -0.55714286 -0.54285714 -0.52857143 -0.51428571 -0.5 -0.48571429 -0.47142857 -0.45714286 -0.44285714 -0.42857143 -0.41428571 -0.4 -0.38571429 -0.37142857 -0.35714286 -0.34285714 -0.32857143 -0.31428571 -0.3 -0.28571429 -0.27142857 -0.25714286 -0.24285714 -0.22857143 -0.21428571 -0.2 -0.18571429 -0.17142857 -0.15714286 -0.14285714 -0.12857143 -0.11428571 -0.1 -0.08571429 -0.07142857 -0.05714286 -0.04285714 -0.02857143 -0.01428571 0 0 0 0 0 0
  line L11 (-12.3428, -6.7149) -> (-13.1686, -6.3857)
  arc A12 (-13.1686, -6.3857) -> (-12.8848, -5.3266) centre (-17.5834, -4.6352) ccw
  line L12 (-12.8848, -5.3266) -> (-12.0051, -5.4543)
  spline S12 degree 5 poles (-12.0051, -5.4543) (-12.0011, -5.4549) (-11.9932, -5.4559) (-11.9812, -5.4571) (-11.9653, -5.458) (-11.9452, -5.458) (-11.9251, -5.4574) (-11.905, -5.4564) (-11.8848, -5.4551) (-11.8646, -5.4536) (-11.8443, -5.4519) (-11.824, -5.4501) (-11.8038, -5.4479) (-11.7834, -5.4454) (-11.7631, -5.4425) (-11.7427, -5.4393) (-11.7224, -5.4358) (-11.702, -5.4321) (-11.6816, -5.4281) (-11.6612, -5.424) (-11.6408, -5.4197) (-11.6203, -5.4151) (-11.5999, -5.4104) (-11.5795, -5.4054) (-11.559, -5.4002) (-11.5386, -5.3947) (-11.5181, -5.3891) (-11.4977, -5.3833) (-11.4772, -5.3773) (-11.4568, -5.3711) (-11.4363, -5.3647) (-11.4159, -5.3581) (-11.3955, -5.3513) (-11.375, -5.3444) (-11.3546, -5.3372) (-11.3342, -5.3299) (-11.3138, -5.3224) (-11.2934, -5.3148) (-11.273, -5.3069) (-11.2526, -5.2989) (-11.2322, -5.2907) (-11.2119, -5.2824) (-11.1915, -5.2738) (-11.1712, -5.2652) (-11.1509, -5.2563) (-11.1305, -5.2473) (-11.1102, -5.2381) (-11.09, -5.2288) (-11.0697, -5.2193) (-11.0495, -5.2096) (-11.0292, -5.1998) (-11.009, -5.1898) (-10.9888, -5.1797) (-10.9687, -5.1694) (-10.9485, -5.1589) (-10.9284, -5.1483) (-10.9083, -5.1376) (-10.8882, -5.1267) (-10.8682, -5.1156) (-10.8481, -5.1044) (-10.8281, -5.0931) (-10.8082, -5.0816) (-10.7882, -5.07) (-10.7683, -5.0582) (-10.7484, -5.0462) (-10.7285, -5.0341) (-10.7087, -5.0219) (-10.6889, -5.0095) (-10.6691, -4.997) (-10.6493, -4.9844) (-10.6296, -4.9716) (-10.6139, -4.9612) (-10.6021, -4.9534) (-10.5942, -4.9482) (-10.5903, -4.9455) knots 0 0 0 0 0 0 0.01428571 0.02857143 0.04285714 0.05714286 0.07142857 0.08571429 0.1 0.11428571 0.12857143 0.14285714 0.15714286 0.17142857 0.18571429 0.2 0.21428571 0.22857143 0.24285714 0.25714286 0.27142857 0.28571429 0.3 0.31428571 0.32857143 0.34285714 0.35714286 0.37142857 0.38571429 0.4 0.41428571 0.42857143 0.44285714 0.45714286 0.47142857 0.48571429 0.5 0.51428571 0.52857143 0.54285714 0.55714286 0.57142857 0.58571429 0.6 0.61428571 0.62857143 0.64285714 0.65714286 0.67142857 0.68571429 0.7 0.71428571 0.72857143 0.74285714 0.75714286 0.77142857 0.78571429 0.8 0.81428571 0.82857143 0.84285714 0.85714286 0.87142857 0.88571429 0.9 0.91428571 0.92857143 0.94285714 0.95714286 0.97142857 0.98571429 1 1 1 1 1 1
  arc A13 (-10.5903, -4.9455) -> (-10.5903, -4.3248) centre (-17.5834, -4.6352) ccw
  spline S13 degree 5 poles (-10.5903, -4.3248) (-10.5942, -4.3222) (-10.6021, -4.317) (-10.6139, -4.3091) (-10.6296, -4.2988) (-10.6493, -4.286) (-10.6691, -4.2733) (-10.6889, -4.2608) (-10.7087, -4.2484) (-10.7285, -4.2362) (-10.7484, -4.2241) (-10.7683, -4.2122) (-10.7882, -4.2004) (-10.8082, -4.1887) (-10.8281, -4.1772) (-10.8481, -4.1659) (-10.8682, -4.1547) (-10.8882, -4.1436) (-10.9083, -4.1327) (-10.9284, -4.122) (-10.9485, -4.1114) (-10.9687, -4.101) (-10.9888, -4.0907) (-11.009, -4.0805) (-11.0292, -4.0706) (-11.0495, -4.0607) (-11.0697, -4.0511) (-11.09, -4.0416) (-11.1102, -4.0322) (-11.1305, -4.0231) (-11.1509, -4.014) (-11.1712, -4.0052) (-11.1915, -3.9965) (-11.2119, -3.988) (-11.2322, -3.9796) (-11.2526, -3.9714) (-11.273, -3.9634) (-11.2934, -3.9556) (-11.3138, -3.9479) (-11.3342, -3.9404) (-11.3546, -3.9331) (-11.375, -3.926) (-11.3955, -3.919) (-11.4159, -3.9123) (-11.4363, -3.9057) (-11.4568, -3.8993) (-11.4772, -3.8931) (-11.4977, -3.8871) (-11.5181, -3.8812) (-11.5386, -3.8756) (-11.559, -3.8702) (-11.5795, -3.865) (-11.5999, -3.86) (-11.6203, -3.8552) (-11.6408, -3.8507) (-11.6612, -3.8464) (-11.6816, -3.8422) (-11.702, -3.8383) (-11.7224, -3.8346) (-11.7427, -3.8311) (-11.7631, -3.8279) (-11.7834, -3.825) (-11.8038, -3.8225) (-11.824, -3.8203) (-11.8443, -3.8184) (-11.8646, -3.8168) (-11.8848, -3.8153) (-11.905, -3.814) (-11.9251, -3.8129) (-11.9452, -3.8123) (-11.9653, -3.8124) (-11.9812, -3.8132) (-11.9932, -3.8144) (-12.0011, -3.8154) (-12.0051, -3.816) knots -1 -1 -1 -1 -1 -1 -0.98571429 -0.97142857 -0.95714286 -0.94285714 -0.92857143 -0.91428571 -0.9 -0.88571429 -0.87142857 -0.85714286 -0.84285714 -0.82857143 -0.81428571 -0.8 -0.78571429 -0.77142857 -0.75714286 -0.74285714 -0.72857143 -0.71428571 -0.7 -0.68571429 -0.67142857 -0.65714286 -0.64285714 -0.62857143 -0.61428571 -0.6 -0.58571429 -0.57142857 -0.55714286 -0.54285714 -0.52857143 -0.51428571 -0.5 -0.48571429 -0.47142857 -0.45714286 -0.44285714 -0.42857143 -0.41428571 -0.4 -0.38571429 -0.37142857 -0.35714286 -0.34285714 -0.32857143 -0.31428571 -0.3 -0.28571429 -0.27142857 -0.25714286 -0.24285714 -0.22857143 -0.21428571 -0.2 -0.18571429 -0.17142857 -0.15714286 -0.14285714 -0.12857143 -0.11428571 -0.1 -0.08571429 -0.07142857 -0.05714286 -0.04285714 -0.02857143 -0.01428571 0 0 0 0 0 0
  line L13 (-12.0051, -3.816) -> (-12.8848, -3.9438)
  arc A14 (-12.8848, -3.9438) -> (-13.1686, -2.8847) centre (-17.5834, -4.6352) ccw
  line L14 (-13.1686, -2.8847) -> (-12.3428, -2.5554)
  spline S14 degree 5 poles (-12.3428, -2.5554) (-12.3391, -2.5539) (-12.3317, -2.5509) (-12.3208, -2.5459) (-12.3066, -2.5387) (-12.2892, -2.5287) (-12.2721, -2.5181) (-12.2551, -2.5071) (-12.2383, -2.4959) (-12.2215, -2.4845) (-12.2048, -2.473) (-12.1882, -2.4612) (-12.1717, -2.4492) (-12.1554, -2.4368) (-12.1392, -2.4242) (-12.1232, -2.4112) (-12.1073, -2.398) (-12.0915, -2.3846) (-12.0758, -2.371) (-12.0602, -2.3572) (-12.0447, -2.3432) (-12.0293, -2.3291) (-12.0139, -2.3148) (-11.9987, -2.3002) (-11.9836, -2.2855) (-11.9686, -2.2706) (-11.9538, -2.2555) (-11.939, -2.2402) (-11.9243, -2.2248) (-11.9097, -2.2092) (-11.8952, -2.1934) (-11.8807, -2.1775) (-11.8664, -2.1614) (-11.8522, -2.1452) (-11.8381, -2.1288) (-11.8241, -2.1122) (-11.8101, -2.0956) (-11.7963, -2.0787) (-11.7825, -2.0617) (-11.7689, -2.0446) (-11.7553, -2.0273) (-11.7419, -2.0099) (-11.7285, -1.9923) (-11.7153, -1.9747) (-11.7021, -1.9568) (-11.689, -1.9389) (-11.676, -1.9208) (-11.6631, -1.9025) (-11.6503, -1.8842) (-11.6376, -1.8657) (-11.625, -1.8471) (-11.6125, -1.8283) (-11.6001, -1.8095) (-11.5878, -1.7905) (-11.5756, -1.7713) (-11.5634, -1.7521) (-11.5514, -1.7328) (-11.5395, -1.7133) (-11.5276, -1.6937) (-11.5159, -1.674) (-11.5042, -1.6541) (-11.4927, -1.6342) (-11.4812, -1.6141) (-11.4698, -1.5939) (-11.4586, -1.5737) (-11.4474, -1.5533) (-11.4363, -1.5327) (-11.4254, -1.5121) (-11.4145, -1.4914) (-11.4037, -1.4706) (-11.393, -1.4496) (-11.3846, -1.4328) (-11.3783, -1.4201) (-11.3741, -1.4116) (-11.372, -1.4074) knots 0 0 0 0 0 0 0.01428571 0.02857143 0.04285714 0.05714286 0.07142857 0.08571429 0.1 0.11428571 0.12857143 0.14285714 0.15714286 0.17142857 0.18571429 0.2 0.21428571 0.22857143 0.24285714 0.25714286 0.27142857 0.28571429 0.3 0.31428571 0.32857143 0.34285714 0.35714286 0.37142857 0.38571429 0.4 0.41428571 0.42857143 0.44285714 0.45714286 0.47142857 0.48571429 0.5 0.51428571 0.52857143 0.54285714 0.55714286 0.57142857 0.58571429 0.6 0.61428571 0.62857143 0.64285714 0.65714286 0.67142857 0.68571429 0.7 0.71428571 0.72857143 0.74285714 0.75714286 0.77142857 0.78571429 0.8 0.81428571 0.82857143 0.84285714 0.85714286 0.87142857 0.88571429 0.9 0.91428571 0.92857143 0.94285714 0.95714286 0.97142857 0.98571429 1 1 1 1 1 1
  arc A15 (-11.372, -1.4074) -> (-11.6823, -0.8698) centre (-17.5834, -4.6352) ccw
  spline S15 degree 5 poles (-11.6823, -0.8698) (-11.6871, -0.8695) (-11.6965, -0.8689) (-11.7106, -0.868) (-11.7294, -0.867) (-11.7529, -0.8657) (-11.7763, -0.8646) (-11.7997, -0.8637) (-11.8231, -0.8629) (-11.8464, -0.8622) (-11.8696, -0.8617) (-11.8928, -0.8613) (-11.916, -0.8611) (-11.9391, -0.8609) (-11.9621, -0.861) (-11.9851, -0.8612) (-12.0081, -0.8615) (-12.031, -0.8619) (-12.0538, -0.8625) (-12.0766, -0.8633) (-12.0993, -0.8642) (-12.122, -0.8652) (-12.1446, -0.8664) (-12.1671, -0.8677) (-12.1896, -0.8691) (-12.2121, -0.8707) (-12.2344, -0.8725) (-12.2567, -0.8744) (-12.279, -0.8765) (-12.3011, -0.8786) (-12.3232, -0.881) (-12.3452, -0.8835) (-12.3672, -0.8861) (-12.3891, -0.8889) (-12.4109, -0.8919) (-12.4326, -0.895) (-12.4543, -0.8982) (-12.4759, -0.9016) (-12.4974, -0.9052) (-12.5188, -0.9089) (-12.5401, -0.9128) (-12.5614, -0.9168) (-12.5826, -0.921) (-12.6036, -0.9254) (-12.6246, -0.9299) (-12.6455, -0.9346) (-12.6663, -0.9394) (-12.6871, -0.9444) (-12.7077, -0.9496) (-12.7282, -0.955) (-12.7486, -0.9605) (-12.7689, -0.9662) (-12.7891, -0.9721) (-12.8092, -0.9782) (-12.8292, -0.9845) (-12.849, -0.9909) (-12.8687, -0.9976) (-12.8884, -1.0043) (-12.9079, -1.0113) (-12.9273, -1.0185) (-12.9465, -1.0259) (-12.9656, -1.0336) (-12.9844, -1.0415) (-13.0031, -1.0498) (-13.0216, -1.0583) (-13.0399, -1.067) (-13.0582, -1.0758) (-13.0763, -1.0848) (-13.0943, -1.094) (-13.112, -1.1035) (-13.1293, -1.1136) (-13.1427, -1.1223) (-13.1525, -1.1293) (-13.1588, -1.1341) (-13.162, -1.1366) knots -1 -1 -1 -1 -1 -1 -0.98571429 -0.97142857 -0.95714286 -0.94285714 -0.92857143 -0.91428571 -0.9 -0.88571429 -0.87142857 -0.85714286 -0.84285714 -0.82857143 -0.81428571 -0.8 -0.78571429 -0.77142857 -0.75714286 -0.74285714 -0.72857143 -0.71428571 -0.7 -0.68571429 -0.67142857 -0.65714286 -0.64285714 -0.62857143 -0.61428571 -0.6 -0.58571429 -0.57142857 -0.55714286 -0.54285714 -0.52857143 -0.51428571 -0.5 -0.48571429 -0.47142857 -0.45714286 -0.44285714 -0.42857143 -0.41428571 -0.4 -0.38571429 -0.37142857 -0.35714286 -0.34285714 -0.32857143 -0.31428571 -0.3 -0.28571429 -0.27142857 -0.25714286 -0.24285714 -0.22857143 -0.21428571 -0.2 -0.18571429 -0.17142857 -0.15714286 -0.14285714 -0.12857143 -0.11428571 -0.1 -0.08571429 -0.07142857 -0.05714286 -0.04285714 -0.02857143 -0.01428571 0 0 0 0 0 0
  line L15 (-13.162, -1.1366) -> (-13.86, -1.6871)
  arc A16 (-13.86, -1.6871) -> (-14.6353, -0.9118) centre (-17.5834, -4.6352) ccw
  line L16 (-14.6353, -0.9118) -> (-14.0848, -0.2138)
  spline S16 degree 5 poles (-14.0848, -0.2138) (-14.0823, -0.2106) (-14.0775, -0.2043) (-14.0705, -0.1945) (-14.0618, -0.1811) (-14.0517, -0.1638) (-14.0422, -0.1461) (-14.033, -0.1281) (-14.024, -0.11) (-14.0152, -0.0917) (-14.0065, -0.0734) (-13.998, -0.0549) (-13.9897, -0.0362) (-13.9818, -0.0174) (-13.9741, 0.0017) (-13.9667, 0.0209) (-13.9595, 0.0403) (-13.9526, 0.0598) (-13.9458, 0.0795) (-13.9391, 0.0992) (-13.9327, 0.119) (-13.9264, 0.139) (-13.9203, 0.1591) (-13.9144, 0.1793) (-13.9087, 0.1996) (-13.9032, 0.22) (-13.8978, 0.2405) (-13.8927, 0.2611) (-13.8876, 0.2819) (-13.8828, 0.3027) (-13.8781, 0.3236) (-13.8736, 0.3446) (-13.8692, 0.3656) (-13.865, 0.3868) (-13.861, 0.4081) (-13.8571, 0.4294) (-13.8534, 0.4508) (-13.8498, 0.4723) (-13.8464, 0.4939) (-13.8432, 0.5156) (-13.8401, 0.5373) (-13.8371, 0.5591) (-13.8343, 0.581) (-13.8317, 0.603) (-13.8292, 0.625) (-13.8269, 0.6471) (-13.8247, 0.6693) (-13.8226, 0.6915) (-13.8207, 0.7138) (-13.819, 0.7361) (-13.8173, 0.7586) (-13.8159, 0.7811) (-13.8146, 0.8036) (-13.8134, 0.8262) (-13.8124, 0.8489) (-13.8115, 0.8716) (-13.8107, 0.8944) (-13.8101, 0.9172) (-13.8097, 0.9401) (-13.8094, 0.9631) (-13.8092, 0.9861) (-13.8092, 1.0091) (-13.8093, 1.0322) (-13.8095, 1.0554) (-13.8099, 1.0786) (-13.8104, 1.1018) (-13.8111, 1.1251) (-13.8119, 1.1485) (-13.8129, 1.1719) (-13.8139, 1.1953) (-13.8152, 1.2188) (-13.8162, 1.2376) (-13.8171, 1.2517) (-13.8177, 1.2612) (-13.8181, 1.2659) knots 0 0 0 0 0 0 0.01428571 0.02857143 0.04285714 0.05714286 0.07142857 0.08571429 0.1 0.11428571 0.12857143 0.14285714 0.15714286 0.17142857 0.18571429 0.2 0.21428571 0.22857143 0.24285714 0.25714286 0.27142857 0.28571429 0.3 0.31428571 0.32857143 0.34285714 0.35714286 0.37142857 0.38571429 0.4 0.41428571 0.42857143 0.44285714 0.45714286 0.47142857 0.48571429 0.5 0.51428571 0.52857143 0.54285714 0.55714286 0.57142857 0.58571429 0.6 0.61428571 0.62857143 0.64285714 0.65714286 0.67142857 0.68571429 0.7 0.71428571 0.72857143 0.74285714 0.75714286 0.77142857 0.78571429 0.8 0.81428571 0.82857143 0.84285714 0.85714286 0.87142857 0.88571429 0.9 0.91428571 0.92857143 0.94285714 0.95714286 0.97142857 0.98571429 1 1 1 1 1 1
  arc A17 (-13.8181, 1.2659) -> (-14.3556, 1.5762) centre (-17.5834, -4.6352) ccw
  spline S17 degree 5 poles (-14.3556, 1.5762) (-14.3598, 1.5741) (-14.3683, 1.5699) (-14.381, 1.5636) (-14.3978, 1.5552) (-14.4188, 1.5445) (-14.4396, 1.5337) (-14.4603, 1.5228) (-14.481, 1.5119) (-14.5015, 1.5008) (-14.5219, 1.4896) (-14.5422, 1.4784) (-14.5623, 1.467) (-14.5824, 1.4556) (-14.6023, 1.444) (-14.6222, 1.4323) (-14.6419, 1.4206) (-14.6615, 1.4088) (-14.681, 1.3968) (-14.7003, 1.3848) (-14.7196, 1.3727) (-14.7387, 1.3604) (-14.7577, 1.3481) (-14.7765, 1.3357) (-14.7953, 1.3232) (-14.8139, 1.3106) (-14.8324, 1.2979) (-14.8507, 1.2851) (-14.869, 1.2722) (-14.8871, 1.2592) (-14.905, 1.2461) (-14.9229, 1.233) (-14.9406, 1.2197) (-14.9581, 1.2063) (-14.9755, 1.1929) (-14.9928, 1.1793) (-15.0099, 1.1657) (-15.0269, 1.1519) (-15.0438, 1.1381) (-15.0605, 1.1242) (-15.077, 1.1101) (-15.0934, 1.096) (-15.1096, 1.0818) (-15.1257, 1.0675) (-15.1416, 1.0531) (-15.1574, 1.0385) (-15.173, 1.0239) (-15.1884, 1.0092) (-15.2037, 0.9945) (-15.2188, 0.9796) (-15.2337, 0.9646) (-15.2484, 0.9495) (-15.263, 0.9343) (-15.2773, 0.919) (-15.2915, 0.9035) (-15.3054, 0.888) (-15.3192, 0.8724) (-15.3328, 0.8567) (-15.3462, 0.8409) (-15.3594, 0.825) (-15.3724, 0.809) (-15.385, 0.7928) (-15.3974, 0.7765) (-15.4094, 0.76) (-15.4212, 0.7434) (-15.4327, 0.7267) (-15.4441, 0.7099) (-15.4554, 0.6931) (-15.4663, 0.6761) (-15.4769, 0.659) (-15.4869, 0.6416) (-15.4941, 0.6274) (-15.4991, 0.6165) (-15.5021, 0.6091) (-15.5036, 0.6054) knots -1 -1 -1 -1 -1 -1 -0.98571429 -0.97142857 -0.95714286 -0.94285714 -0.92857143 -0.91428571 -0.9 -0.88571429 -0.87142857 -0.85714286 -0.84285714 -0.82857143 -0.81428571 -0.8 -0.78571429 -0.77142857 -0.75714286 -0.74285714 -0.72857143 -0.71428571 -0.7 -0.68571429 -0.67142857 -0.65714286 -0.64285714 -0.62857143 -0.61428571 -0.6 -0.58571429 -0.57142857 -0.55714286 -0.54285714 -0.52857143 -0.51428571 -0.5 -0.48571429 -0.47142857 -0.45714286 -0.44285714 -0.42857143 -0.41428571 -0.4 -0.38571429 -0.37142857 -0.35714286 -0.34285714 -0.32857143 -0.31428571 -0.3 -0.28571429 -0.27142857 -0.25714286 -0.24285714 -0.22857143 -0.21428571 -0.2 -0.18571429 -0.17142857 -0.15714286 -0.14285714 -0.12857143 -0.11428571 -0.1 -0.08571429 -0.07142857 -0.05714286 -0.04285714 -0.02857143 -0.01428571 0 0 0 0 0 0
  line L17 (-15.5036, 0.6054) -> (-15.8329, -0.2204)
  arc A18 (-15.8329, -0.2204) -> (-16.892, 0.0634) centre (-17.5834, -4.6352) ccw
  line L18 (-16.892, 0.0634) -> (-16.7642, 0.9432)
  spline S18 degree 5 poles (-16.7642, 0.9432) (-16.7637, 0.9471) (-16.7626, 0.955) (-16.7615, 0.967) (-16.7606, 0.9829) (-16.7605, 1.003) (-16.7611, 1.0231) (-16.7622, 1.0432) (-16.7635, 1.0634) (-16.765, 1.0837) (-16.7666, 1.1039) (-16.7685, 1.1242) (-16.7707, 1.1445) (-16.7732, 1.1648) (-16.7761, 1.1851) (-16.7793, 1.2055) (-16.7828, 1.2258) (-16.7865, 1.2462) (-16.7904, 1.2666) (-16.7946, 1.287) (-16.7989, 1.3075) (-16.8034, 1.3279) (-16.8082, 1.3483) (-16.8132, 1.3687) (-16.8184, 1.3892) (-16.8238, 1.4096) (-16.8294, 1.4301) (-16.8353, 1.4505) (-16.8413, 1.471) (-16.8475, 1.4914) (-16.8539, 1.5119) (-16.8605, 1.5323) (-16.8672, 1.5527) (-16.8742, 1.5732) (-16.8813, 1.5936) (-16.8886, 1.614) (-16.8961, 1.6344) (-16.9038, 1.6548) (-16.9116, 1.6752) (-16.9197, 1.6956) (-16.9278, 1.716) (-16.9362, 1.7363) (-16.9447, 1.7567) (-16.9534, 1.777) (-16.9623, 1.7974) (-16.9713, 1.8177) (-16.9804, 1.838) (-16.9898, 1.8582) (-16.9993, 1.8785) (-17.009, 1.8987) (-17.0188, 1.919) (-17.0288, 1.9392) (-17.0389, 1.9594) (-17.0492, 1.9795) (-17.0596, 1.9997) (-17.0702, 2.0198) (-17.081, 2.0399) (-17.0919, 2.06) (-17.1029, 2.08) (-17.1141, 2.1001) (-17.1255, 2.1201) (-17.137, 2.14) (-17.1486, 2.16) (-17.1604, 2.1799) (-17.1723, 2.1998) (-17.1844, 2.2197) (-17.1966, 2.2395) (-17.209, 2.2593) (-17.2215, 2.2791) (-17.2342, 2.2989) (-17.247, 2.3186) (-17.2573, 2.3344) (-17.2652, 2.3462) (-17.2704, 2.354) (-17.273, 2.3579) knots 0 0 0 0 0 0 0.01428571 0.02857143 0.04285714 0.05714286 0.07142857 0.08571429 0.1 0.11428571 0.12857143 0.14285714 0.15714286 0.17142857 0.18571429 0.2 0.21428571 0.22857143 0.24285714 0.25714286 0.27142857 0.28571429 0.3 0.31428571 0.32857143 0.34285714 0.35714286 0.37142857 0.38571429 0.4 0.41428571 0.42857143 0.44285714 0.45714286 0.47142857 0.48571429 0.5 0.51428571 0.52857143 0.54285714 0.55714286 0.57142857 0.58571429 0.6 0.61428571 0.62857143 0.64285714 0.65714286 0.67142857 0.68571429 0.7 0.71428571 0.72857143 0.74285714 0.75714286 0.77142857 0.78571429 0.8 0.81428571 0.82857143 0.84285714 0.85714286 0.87142857 0.88571429 0.9 0.91428571 0.92857143 0.94285714 0.95714286 0.97142857 0.98571429 1 1 1 1 1 1
  arc A19 (-17.273, 2.3579) -> (-17.8937, 2.3579) centre (-17.5834, -4.6352) ccw
  spline S19 degree 5 poles (-17.8937, 2.3579) (-17.8964, 2.354) (-17.9016, 2.3462) (-17.9094, 2.3344) (-17.9198, 2.3186) (-17.9326, 2.2989) (-17.9452, 2.2791) (-17.9578, 2.2593) (-17.9701, 2.2395) (-17.9824, 2.2197) (-17.9944, 2.1998) (-18.0064, 2.1799) (-18.0182, 2.16) (-18.0298, 2.14) (-18.0413, 2.1201) (-18.0527, 2.1001) (-18.0639, 2.08) (-18.0749, 2.06) (-18.0858, 2.0399) (-18.0966, 2.0198) (-18.1072, 1.9997) (-18.1176, 1.9795) (-18.1279, 1.9594) (-18.138, 1.9392) (-18.148, 1.919) (-18.1578, 1.8987) (-18.1675, 1.8785) (-18.177, 1.8582) (-18.1863, 1.838) (-18.1955, 1.8177) (-18.2045, 1.7974) (-18.2134, 1.777) (-18.2221, 1.7567) (-18.2306, 1.7363) (-18.2389, 1.716) (-18.2471, 1.6956) (-18.2551, 1.6752) (-18.263, 1.6548) (-18.2706, 1.6344) (-18.2781, 1.614) (-18.2854, 1.5936) (-18.2926, 1.5732) (-18.2995, 1.5527) (-18.3063, 1.5323) (-18.3129, 1.5119) (-18.3193, 1.4914) (-18.3255, 1.471) (-18.3315, 1.4505) (-18.3373, 1.4301) (-18.343, 1.4096) (-18.3484, 1.3892) (-18.3536, 1.3687) (-18.3586, 1.3483) (-18.3633, 1.3279) (-18.3679, 1.3075) (-18.3722, 1.287) (-18.3763, 1.2666) (-18.3803, 1.2462) (-18.384, 1.2258) (-18.3875, 1.2055) (-18.3907, 1.1851) (-18.3936, 1.1648) (-18.3961, 1.1445) (-18.3983, 1.1242) (-18.4001, 1.1039) (-18.4018, 1.0837) (-18.4033, 1.0634) (-18.4046, 1.0432) (-18.4056, 1.0231) (-18.4063, 1.003) (-18.4062, 0.9829) (-18.4053, 0.967) (-18.4041, 0.955) (-18.4031, 0.9471) (-18.4025, 0.9432) knots -1 -1 -1 -1 -1 -1 -0.98571429 -0.97142857 -0.95714286 -0.94285714 -0.92857143 -0.91428571 -0.9 -0.88571429 -0.87142857 -0.85714286 -0.84285714 -0.82857143 -0.81428571 -0.8 -0.78571429 -0.77142857 -0.75714286 -0.74285714 -0.72857143 -0.71428571 -0.7 -0.68571429 -0.67142857 -0.65714286 -0.64285714 -0.62857143 -0.61428571 -0.6 -0.58571429 -0.57142857 -0.55714286 -0.54285714 -0.52857143 -0.51428571 -0.5 -0.48571429 -0.47142857 -0.45714286 -0.44285714 -0.42857143 -0.41428571 -0.4 -0.38571429 -0.37142857 -0.35714286 -0.34285714 -0.32857143 -0.31428571 -0.3 -0.28571429 -0.27142857 -0.25714286 -0.24285714 -0.22857143 -0.21428571 -0.2 -0.18571429 -0.17142857 -0.15714286 -0.14285714 -0.12857143 -0.11428571 -0.1 -0.08571429 -0.07142857 -0.05714286 -0.04285714 -0.02857143 -0.01428571 0 0 0 0 0 0
  line L19 (-18.4025, 0.9432) -> (-18.2748, 0.0634)
  arc A20 (-18.2748, 0.0634) -> (-19.3339, -0.2204) centre (-17.5834, -4.6352) ccw
  line L20 (-19.3339, -0.2204) -> (-19.6631, 0.6054)